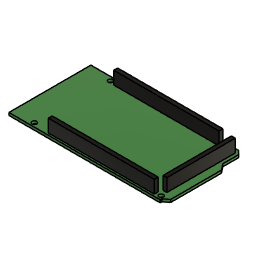
Mega (Autodesk Fusion 360 design; units mm, degrees)
Autodesk Fusion 360 part; units mm, degrees
sketch "Boceto1" plane through (0, 0, 0) normal (0, 0, 1) x (1, 0, 0)
  line L0 (-50.8, 26.67) -> (50.8, 26.67)
  line L1 (50.8, 26.67) -> (50.8, -26.67)
  line L2 (50.8, -26.67) -> (-50.8, -26.67)
  line L3 (-50.8, -26.67) -> (-50.8, 26.67)
  line L4 (-50.8, 0) -> (50.8, 0) construction
  circle A0 centre (-35.56, 24.13) radius 1.5
  circle A1 centre (39.37, 24.13) radius 1.5
  circle A2 centre (45.72, -24.13) radius 1.5
  circle A3 centre (-36.83, -24.13) radius 1.5
  circle A4 centre (15.24, -19.05) radius 1.5
  line L5 (45.2477, 26.67) -> (47.6517, 24.3349)
  line L6 (47.6517, 24.3349) -> (47.6517, 13.9338)
  line L7 (47.6517, 13.9338) -> (50.8, 10.0089)
  line L8 (47.6442, -26.67) -> (47.6442, -25.5537)
  line L9 (47.6442, -25.5537) -> (50.8, -23.002)
  line L10 (-32.1884, 25.38) -> (36.3857, 25.38)
  line L11 (36.3857, 25.38) -> (36.3857, 22.88)
  line L12 (36.3857, 22.88) -> (-32.1884, 22.88)
  line L13 (-32.1884, 22.88) -> (-32.1884, 25.38)
  line L14 (-32.1884, 25.38) -> (36.3857, 22.88) construction
  line L15 (36.3857, 25.38) -> (-32.1884, 22.88) construction
  line L16 (43.14, 24.13) -> (45.64, 24.13)
  line L17 (45.64, 24.13) -> (45.64, -20.35)
  line L18 (45.64, -20.35) -> (43.14, -20.35)
  line L19 (43.14, -20.35) -> (43.14, 24.13)
  line L20 (43.14, 24.13) -> (45.64, -20.35) construction
  line L21 (45.64, 24.13) -> (43.14, -20.35) construction
  line L22 (-26.4326, -22.88) -> (42.4806, -22.88)
  line L23 (42.4806, -22.88) -> (42.4806, -25.38)
  line L24 (42.4806, -25.38) -> (-26.4326, -25.38)
  line L25 (-26.4326, -25.38) -> (-26.4326, -22.88)
  line L26 (-26.4326, -22.88) -> (42.4806, -25.38) construction
  line L27 (42.4806, -22.88) -> (-26.4326, -25.38) construction
  point P0 (2.0986, 24.13)
  point P1 (44.39, 1.89)
  point P2 (8.024, -24.13)
  dimension "d2" = 53.34
  dimension "d3" = 101.6
  dimension "d4" = 13.97
  dimension "d5" = 15.24
  dimension "d7" = 2.54
  dimension "d8" = 50.8
  dimension "d9" = 96.52
  dimension "d10" = 90.17
  dimension "d11" = 7.62
  dimension "d12" = 66.04
  dimension "d13" = 3
  dimension "d17" = 2.5
  dimension "d18" = 2.5
  dimension "d19" = 2.5
  constraint horizontal L0
  constraint vertical L1
  constraint horizontal L2
  constraint vertical L3
  constraint midpoint L3 L4.start
  constraint midpoint L1 L4.end
  constraint midpoint origin L4
  constraint equal A0 A1
  constraint equal A1 A2
  constraint equal A2 A3
  constraint horizontal A2.centre A3.centre
  constraint horizontal A0.centre A1.centre
  constraint equal A2 A4
  constraint coincident L0 L5.start
  constraint perpendicular L0 L6
  constraint coincident L1 L7.end
  constraint coincident L2 L8.start
  constraint perpendicular L2 L8
  constraint coincident L1 L9.end
  constraint horizontal L10
  constraint perpendicular L10 L11
  constraint parallel L10 L12
  constraint parallel L11 L13
  constraint coincident L14 P0
  constraint coincident L15 P0
  constraint horizontal L16
  constraint perpendicular L16 L17
  constraint parallel L16 L18
  constraint parallel L17 L19
  constraint coincident L20 P1
  constraint coincident L21 P1
  constraint horizontal L22
  constraint perpendicular L22 L23
  constraint parallel L22 L24
  constraint parallel L23 L25
  constraint coincident L26 P2
  constraint coincident L27 P2
  constraint horizontal A0.centre P0
  constraint coincident A1.centre L16
  constraint horizontal A3.centre P2
  measures "d2" distance of L0.end L1.end
  measures "d3" distance of L0.start L0.end
  measures "d4" distance of L3 A3.centre
  measures "d5" distance of L3 A0.centre
  measures "d7" distance of L2 A3.centre
  measures "d8" distance of L2 A0.centre
  measures "d9" distance of L3 A2.centre
  measures "d10" distance of L3 A1.centre
  measures "d11" distance of L2 A4.centre
  measures "d12" distance of L3 A4.centre
  measures "d13" diameter of A0
  measures "d17" distance of L10.end L11.end
  measures "d18" distance of L16.start L16.end
  measures "d19" distance of L22.end L23.end
extrude "Extruir1" add sketch "Boceto1" against normal blind 1.7 contours L0 L1 L2 L3 L5 L6 L7 L8 L9 | L10 L11 L12 L13 | L16 L17 L18 L19 | L22 L23 L24 L25
extrude "Extruir2" add sketch "Boceto1" along normal blind 8.34 contours L10 L11 L12 L13 | L16 L17 L18 L19 | L22 L23 L24 L25
